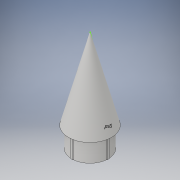
# Autodesk Inventor part: Nose Cone MK I
Saved by Autodesk Inventor 2017 (Build 210142000, 142)
## iProperties
Created: 2017-05-18
Part Number: Nose Cone MK I
Material: Generic
Document SubType Name: Modeling
Designer: Harrison
Density: 1 g/cm^3
Appearance: Default
Author: Harrison
Autodesk Inventor part; units mm, degrees
ref_plane "YZ Plane" through (0, 0, 0) normal (1, 0, 0) x (0, 1, 0)
ref_plane "XZ Plane" through (0, 0, 0) normal (0, 1, 0) x (-1, 0, 0)
ref_plane "XY Plane" through (0, 0, 0) normal (0, 0, 1) x (1, 0, 0)
sketch "Sketch1" plane through (0, 0, 0) normal (1, 0, 0) x (0, 1, 0)
  line L0 (0, -22.86) -> (-25.4, -22.86)
  line L1 (-25.4, -22.86) -> (-25.4, 0)
  line L2 (-25.4, 0) -> (0, 0)
  line L3 (101.6, 0) -> (0, -26.924)
  line L4 (101.6, 0) -> (0, 0)
  line L5 (1.2682, -25.276) -> (91.8637, -1.2682)
  line L6 (-24.13, -21.59) -> (-1.27, -21.59)
  line L7 (-1.27, -21.59) -> (1.2682, -21.59)
  line L8 (-24.13, -21.59) -> (-25.4, -21.59)
  line L9 (91.8637, -1.2682) -> (96.6492, 0)
  line L10 (1.2682, -21.59) -> (1.2682, -25.276)
  line L11 (0, -26.924) -> (0, -22.86)
  dimension "d27" = 1.27
  constraints: 24 end point, 3 perpendicular, 2 point on line, 1 collinear, 1 horizontal, 1 vertical
  measures "d27" distance between parallel lines of L0 L6
revolve "Revolution1" add sketch "Sketch1" angle 360 about axis through (0, 101.6, 0) along (0, -1, 0) contours L0 L1 L8 L6 L7 L10 L5 L9 L4 L3 L11
revolve "Revolution2" add sketch "Sketch1" angle 360 about axis through (0, -25.4, 0) along (0, 1, 0) contours L1 L2 L4 L9 L5 L10 L7 L6 L8
sketch "Sketch2" plane through (0, -25.4, 0) normal (0, -1, 0) x (1, 0, 0)
  line L0 (0, 0) -> (22.86, 0)
  circle A0 centre (0, 0) radius 22.86 projected
  arc A1 (23.1962, -1.5875) -> (23.1962, 1.5875) centre (0, 0) ccw
  line L1 (22.8048, 1.5875) -> (23.1962, 1.5875)
  line L2 (22.8048, -1.5875) -> (23.1962, -1.5875)
  line L3 (0, -22.86) -> (1.5875, -22.86)
  line L4 (0, -22.86) -> (1.5875, -22.86) construction
  line L5 (0, -22.86) -> (-1.5875, -22.86)
  circle A2 centre (0, 0) radius 23.241
  line L6 (-1.5875, -22.8048) -> (-1.5875, -23.1867)
  line L7 (1.5875, -22.8048) -> (1.5875, -23.1867)
  line L8 (-22.86, 0) -> (-22.86, -1.5875)
  line L9 (-22.86, 0) -> (-22.86, 1.5875)
  line L10 (-22.8048, 1.5875) -> (-23.1867, 1.5875)
  line L11 (-22.8048, -1.5875) -> (-23.1867, -1.5875)
  line L12 (0, 22.86) -> (1.5875, 22.86)
  line L13 (0, 22.86) -> (1.5875, 22.86) construction
  line L14 (0, 22.86) -> (-1.5875, 22.86)
  line L15 (0, 22.86) -> (1.5875, 22.86) construction
  line L16 (-1.5875, 22.8048) -> (-1.5875, 23.1867)
  line L17 (1.5875, 22.8048) -> (1.5875, 23.1867)
  dimension "d14" = 1.5875
  dimension "d16" = 1.5875
  dimension "d17" = 0.381
  dimension "d18" = 1.5875
  dimension "d19" = 1.5875
  dimension "d21" = 1.5875
  dimension "d22" = 0
  dimension "d23" = 1.5875
  dimension "d24" = 180
  constraints: 36 end point, 14 horizontal, 8 point on circle, 7 vertical, 3 collinear, 2 centre point, 1 parallel, 1 point on line, 13 other
  measures "d14" distance of L3.start L3.end
  measures "d16" distance of L3.start L5.end
  measures "d18" distance of L8.start L8.end
  measures "d19" distance of L8.start L9.end
  measures "d21" distance of L12.start L12.end
  measures "d22" distance between parallel lines of L12 L13
  measures "d23" distance of L12.start L14.end
  measures "d24" angle of L14 L15
extrude "Extrusion1" add sketch "Sketch2" against normal blind 25.4 contours A0 L1 A2 L2 | A0 L12 L17 | L1 A1 L2 A2 | L7 L3 A0 | L14 L16 A2 L17 L12 | A0 L16 L14 | L5 L6 A0 | L3 L7 A2 L6 L5 | A0 L9 L10 | L10 L9 L8 L11 A2 | L11 L8 A0
revolve "Revolution3" cut sketch "Sketch1" angle 360 about axis through (0, -25.4, 0) along (0, 1, 0) contours L1 L2 L4 L9 L5 L10 L7 L6 L8
revolve "Revolution4" cut sketch "Sketch1" angle 360 about axis through (0, 101.6, 0) along (0, -1, 0) contours L1 L2 L4 L9 L5 L10 L7 L6 L8
body "Solid1"
